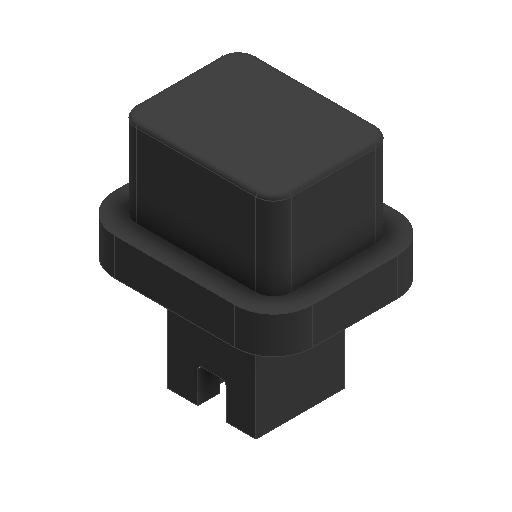
# Autodesk Inventor part: Button_cap_OCP
Saved by Autodesk Inventor 2025 (Build 290162000, 162)
## iProperties
Created: 2025-01-02
Part Number: Button_cap_OCP
Material: Generic
Document SubType Name: Modeling
Designer: Jan Mareš
Density: 1 g/cm^3
Appearance: Default
Author: Jan Mareš
Autodesk Inventor part; units mm, degrees
ref_plane "YZ Plane" through (0, 0, 0) normal (1, 0, 0) x (0, 1, 0)
ref_plane "XZ Plane" through (0, 0, 0) normal (0, 1, 0) x (-1, 0, 0)
ref_plane "XY Plane" through (0, 0, 0) normal (0, 0, 1) x (1, 0, 0)
sketch "Sketch1" plane through (0, 0, 0) normal (0, 1, 0) x (-1, 0, 0)
  line L0 (3.5, 0) -> (-3.5, 0) construction
  line L1 (0, -3.5) -> (0, 3.5) construction
  line L2 (-2.5, 2.5) -> (2.5, 2.5)
  line L3 (2.5, 2.5) -> (2.5, -2.5)
  line L4 (2.5, -2.5) -> (-2.5, -2.5)
  line L5 (-2.5, -2.5) -> (-2.5, 2.5)
  line L6 (-2.5, 0) -> (2.5, 0) construction
  point P0 (0, 0)
  dimension "d0" = 5
  constraints: 10 end point, 3 midpoint, 2 parallel, 2 perpendicular, 1 horizontal
  measures "d0" distance of L2.start L2.end
extrude "Extrusion1" add sketch "Sketch1" along normal blind 6
sketch "Sketch2" plane through (0, 0, 0) normal (0, -1, 0) x (1, 0, 0)
  line L0 (-1.25, 1.25) -> (1.25, 1.25)
  line L1 (1.25, 1.25) -> (1.25, -1.25)
  line L2 (1.25, -1.25) -> (-1.25, -1.25)
  line L3 (-1.25, -1.25) -> (-1.25, 1.25)
  line L4 (-1.25, 0) -> (1.25, 0) construction
  point P0 (0, 0)
  point P1 (0, 0)
  dimension "d3" = 2.5
  constraints: 10 end point, 3 midpoint, 2 parallel, 2 perpendicular, 1 coincident, 1 horizontal
  measures "d3" distance of L0.start L0.end
extrude "Extrusion2" cut sketch "Sketch2" against normal blind 2.8
sketch "Sketch3" plane through (-2.5, 0, 2.5) normal (0, 0, 1) x (1, 0, 0)
  line L0 (2.5, -1.2) -> (2.5, 7.2) construction
  line L1 (-1, 0) -> (6, 0) construction
  line L2 (1.7, 0) -> (1.7, 2)
  line L3 (1.7, 2) -> (3.3, 2)
  line L4 (3.3, 2) -> (3.3, 0)
  line L5 (1.7, 0) -> (3.3, 0)
  line L6 (1.7, 1) -> (3.3, 1) construction
  point P0 (2.5, 0)
  point P1 (2.5, 1)
  dimension "d6" = 1.6
  dimension "d7" = 2
  constraints: 10 end point, 3 midpoint, 3 point on line, 2 perpendicular, 1 collinear, 1 vertical
  measures "d6" distance of L2.end L3.end
  measures "d7" distance of L3.end L4.end
extrude "Extrusion3" cut sketch "Sketch3" against normal through all
sketch "Sketch4" plane through (0, 0, 0) normal (0, 0, 1) x (1, 0, 0)
  line L0 (1.25, 0) -> (1.25, 2.8) construction
  line L1 (-1.25, 0) -> (-1.25, 2.8) construction
  line L2 (-1.758, 0) -> (1.798, 0) construction
  arc A0 (1.25, 0.9) -> (1.25, 0.6317) centre (1.29, 0.7658) ccw
  line L3 (1.29, 0.7658) -> (1.15, 0.7658) construction
  line L4 (1.25, 0.6317) -> (1.25, 0.9) construction
  line L5 (1.1441, 0.9) -> (1.25, 0.9)
  line L6 (1.1441, 0.9) -> (1.25, 0.7165)
  line L7 (1.25, 0.9) -> (1.25, 0.7165)
  line L8 (1.25, 0.9) -> (1.25, 0.6317)
  point P0 (0, 0)
  dimension "d13" = 0.1
  dimension "d14" = 1.9
  dimension "d15" = 0.14
  dimension "d28" = 30
  dimension "d29" = 0.106
  dimension "d30" = 1.9
  constraints: 12 end point, 6 point on line, 3 point on circle, 1 centre point, 1 collinear, 1 horizontal, 1 perpendicular
  measures "d13" distance from line of L0 L3.end
  measures "d14" distance of L4.end L0.end
  measures "d15" radius of A0
  measures "d28" angle of L0 L6
  measures "d29" distance of L5.start L5.end
  measures "d30" distance from line of L5 L0.end
extrude "Extrusion4" add sketch "Sketch4" along normal through all both and the other way through all contours L7 L6 A0 | L6 L8 A0
mirror "Mirror1" about plane through (0, 0, 0) normal (1, 0, 0) of "Extrusion4"
sketch "Sketch5" plane through (0, 6, 0) normal (0, 1, 0) x (1, 0, 0)
  line L0 (-4.4, -3.4) -> (4.4, -3.4)
  line L1 (4.4, -3.4) -> (4.4, 3.4)
  line L2 (4.4, 3.4) -> (-4.4, 3.4)
  line L3 (-4.4, 3.4) -> (-4.4, -3.4)
  line L4 (0, -3.4) -> (0, 3.4) construction
  line L5 (6.16, 0) -> (-6.16, 0) construction
  point P0 (0, 0)
  dimension "d18" = 6.8
  dimension "d19" = 8.8
  constraints: 10 end point, 3 midpoint, 2 parallel, 1 horizontal, 1 perpendicular
  measures "d18" distance of L2.end L0.start
  measures "d19" distance of L0.start L0.end
extrude "Extrusion5" add sketch "Sketch5" along normal blind 7
fillet "Fillet1" radius 1 4 edges at (4.4, 9.5, 3.4) (4.4, 9.5, -3.4) (-4.4, 9.5, 3.4) (-4.4, 9.5, -3.4)
fillet "Fillet2" radius 0.2 8 edges at (4.1071, 13, -3.1071) (0, 13, -3.4) (-4.1071, 13, -3.1071) (-4.4, 13, 0) (-4.1071, 13, 3.1071) (0, 13, 3.4) (4.1071, 13, 3.1071) (4.4, 13, 0)
sketch "Sketch6" plane through (0, 6, 0) normal (0, -1, 0) x (1, 0, 0)
  line L0 (-3.4, 3.4) -> (3.4, 3.4) projected
  arc A0 (4.4, 2.4) -> (3.4, 3.4) centre (3.4, 2.4) ccw projected
  line L1 (4.4, 2.4) -> (4.4, -2.4) projected
  arc A1 (3.4, -3.4) -> (4.4, -2.4) centre (3.4, -2.4) ccw projected
  line L2 (3.4, -3.4) -> (-3.4, -3.4) projected
  arc A2 (-4.4, -2.4) -> (-3.4, -3.4) centre (-3.4, -2.4) ccw projected
  line L3 (-4.4, -2.4) -> (-4.4, 2.4) projected
  arc A3 (-3.4, 3.4) -> (-4.4, 2.4) centre (-3.4, 2.4) ccw projected
  line L4 (3.4, 4.6) -> (-3.4, 4.6)
  arc A4 (-3.4, 4.6) -> (-5.6, 2.4) centre (-3.4, 2.4) ccw
  line L5 (-5.6, 2.4) -> (-5.6, -2.4)
  arc A5 (-5.6, -2.4) -> (-3.4, -4.6) centre (-3.4, -2.4) ccw
  line L6 (-3.4, -4.6) -> (3.4, -4.6)
  arc A6 (3.4, -4.6) -> (5.6, -2.4) centre (3.4, -2.4) ccw
  line L7 (5.6, -2.4) -> (5.6, 2.4)
  arc A7 (5.6, 2.4) -> (3.4, 4.6) centre (3.4, 2.4) ccw
  point P0 (0, 0)
  dimension "d24" = 1.2
  constraints: 8 end point, 8 point on circle, 4 centre point, 7 other
  measures "d24" distance between parallel lines of L0 L4
extrude "Extrusion6" add sketch "Sketch6" against normal blind 2.1
fillet "Fillet3" radius 0.6 4 edges at (0, 6, 2.5) (-2.5, 6, 0) (2.5, 6, 0) (0, 6, -2.5)
fillet "Fillet4" radius 0.2 4 edges at (0, 2.8, 1.25) (-1.25, 2.8, 0) (0, 2.8, -1.25) (1.25, 2.8, 0)
fillet "Fillet5" radius 0.2 4 edges at (0.8, 2, 1.875) (-0.8, 2, 1.875) (-0.8, 2, -1.875) (0.8, 2, -1.875)
ref_plane "Work Plane1" through (0, 0, 0) normal (1, 0, 0) x (0, 1, 0)
body "Solid1"
